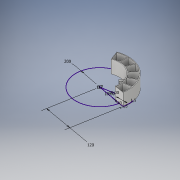
# Autodesk Inventor part: bacRecupBonbon
Saved by Autodesk Inventor 2019 (Build 230136000, 136)
## iProperties
Created: 2021-01-08
Part Number: bacRecupBonbon
Material: Générique
Document SubType Name: Modeling
Designer: tom.mousset
Density: 1 g/cm^3
Appearance: Par défaut
Author: tom.mousset
## iProperties of the stored document BVav_Impression 3D.ipt
Created: 2021-01-08
Part Number: BVav_Impression 3D
Material: Générique
Document SubType Name: Modeling
Designer: tom.mousset
Density: 1 g/cm^3
Appearance: Par défaut
Author: tom.mousset
Autodesk Inventor part; units mm, degrees
ref_plane "YZ Plane" through (0, 0, 0) normal (1, 0, 0) x (0, 1, 0)
ref_plane "XZ Plane" through (0, 0, 0) normal (0, 1, 0) x (-1, 0, 0)
sketch "Esquisse1" plane through (0, 0, 0) normal (0, 1, 0) x (-1, 0, 0)
  circle A0 centre (0, 0) radius 100
  line L0 (0, 0) -> (-118.1769, 20.8378)
  line L1 (0, 0) -> (-2.1593, 0)
  line L2 (0, 0) -> (-118.1769, -20.8378)
  arc A1 (-118.1769, 20.8378) -> (-118.1769, -20.8378) centre (0, 0) ccw
  line L3 (-118.1769, 20.8378) -> (-78.7846, 13.8919)
  arc A2 (-78.7846, 13.8919) -> (-78.7846, -13.8919) centre (0, 0) ccw
  line L4 (-78.7846, -13.8919) -> (-118.1769, -20.8378)
  arc A3 (-115.2225, 20.3168) -> (-115.2225, -20.3168) centre (0, 0) ccw
  arc A4 (-81.739, 14.4128) -> (-81.739, -14.4128) centre (0, 0) ccw
  line L5 (-115.4735, 18.838) -> (-81.9862, 12.9332)
  line L6 (-115.4735, -18.838) -> (-81.9862, -12.9332)
  dimension "d0" = 200
  dimension "d1" = 10
  dimension "d2" = 10
  dimension "d3" = 40
  dimension "d4" = 120
  dimension "d5" = 117
  dimension "d6" = 83
  dimension "d7" = 1.5
  dimension "d8" = 1.5
  constraints: 14 end point, 12 point on circle, 7 point on line, 5 centre point, 5 coincident, 2 parallel, 1 collinear, 1 equal length, 1 horizontal
  measures "d0" diameter of A0
  measures "d1" angle of L0 L1
  measures "d2" angle of L1 L2
  measures "d3" distance of L0.end L3.end
  measures "d4" distance of L0.start L0.end
  measures "d5" radius of A3
  measures "d6" radius of A4
  measures "d7" distance between parallel lines of L3 L5
  measures "d8" distance between parallel lines of L2 L6
extrude "Extrusion2" add sketch "Esquisse1" along normal blind 50 and the other way blind 3.5 contours L0 A4 L5 A0 | A0 L5 A3 L0 | L2 A3 L6 A0 | A0 L6 A4 L2 | L5 A4 L6 A0 | A0 L6 A3 L5 | L0 A2 L2 A4 | A3 L2 A1 L0
extrude "Extrusion3" cut sketch "Esquisse1" along normal blind 60 contours L5 A4 L6 A0 | A0 L6 A3 L5
pattern_circular "Réseau circulaire1" count 6 over 100 about axis through (0, -10, 0) along (0, 1, 0) of "Extrusion2", "Extrusion3"
sketch "Esquisse2" plane through (0, -3.5, 0) normal (0, -1, 0) x (1, 0, 0)
  line L0 (0, 0) -> (51.423, -61.2836)
  arc A0 (-27.3616, -75.1754) -> (78.7846, 13.8919) centre (0, 0) ccw projected
  line L1 (0, 0) -> (78.7846, 13.8919)
  line L2 (62.0017, -50.5549) -> (69.6621, -44.127)
  line L3 (69.6621, -44.127) -> (56.8064, -28.8061)
  line L4 (56.8064, -28.8061) -> (49.1459, -35.234)
  line L5 (49.1459, -35.234) -> (62.0017, -50.5549)
  dimension "d20" = 60
  dimension "d21" = 10
  dimension "d22" = 15
  dimension "d23" = 20
  constraints: 12 end point, 2 parallel, 2 perpendicular, 2 point on circle
  measures "d20" angle of L1 L0
  measures "d21" distance of L2.start L2.end
  measures "d22" distance from line of L0 L2.start
  measures "d23" distance of L4.end L2.start
extrude "Extrusion4" add sketch "Esquisse2" against normal blind 10 contours L5 L4 L3 A0 | A0 L3 L2
ref_plane "Plan de construction1" through (0, 0, 0) normal (0.766, 0, 0.6428) x (0.6422, -0.0437, -0.7653)
mirror "Symétrie1" about plane through (0, 0, 0) normal (0.766, 0, 0.6428) of "Extrusion4"
